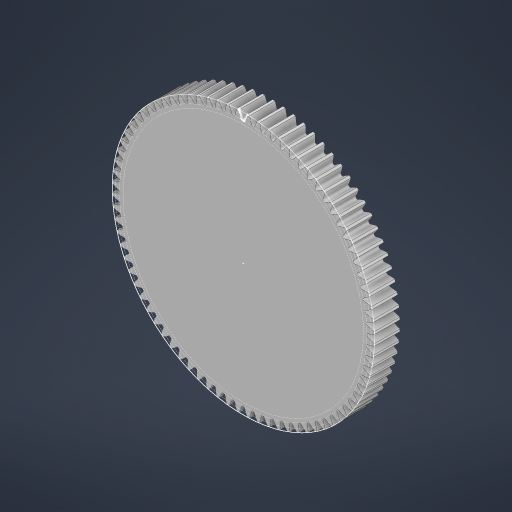
# Autodesk Inventor part: horizontal_axis_hal_gearr
Saved by Autodesk Inventor 2023.2 (Build 272271000, 271)
## iProperties
Created: 2023-07-30
Part Number: horizontal_axis_hal_gearr
Material: Generic
Document SubType Name: Modeling
Designer: Bober
Density: 1 g/cm^3
Appearance: Default
Author: Bober
Autodesk Inventor part; units mm, degrees
ref_plane "YZ Plane" through (0, 0, 0) normal (1, 0, 0) x (0, 1, 0)
ref_plane "XZ Plane" through (0, 0, 0) normal (0, 1, 0) x (-1, 0, 0)
ref_plane "XY Plane" through (0, 0, 0) normal (0, 0, 1) x (1, 0, 0)
sketch "Sketch1" plane through (0, 0, 0) normal (0, 0, 1) x (1, 0, 0)
  spline S0 degree 3 poles (-1.2376, 40.9813) (-1.1892, 40.8773) (-1.0925, 40.6692) (-0.9561, 40.3531) (-0.8267, 40.0342) (-0.7055, 39.712) (-0.5926, 39.3868) (-0.516, 39.1404) (-0.4674, 38.9752) (-0.4334, 38.8959) (-0.3865, 38.8233) (-0.3362, 38.7714) (-0.2894, 38.7381) (-0.2524, 38.7161) (-0.2127, 38.6991) (-0.1714, 38.6872) (-0.1291, 38.6784) (-0.0717, 38.676) (0, 38.6775) (0.0717, 38.676) (0.1291, 38.6784) (0.1714, 38.6872) (0.2127, 38.6991) (0.2524, 38.7161) (0.2894, 38.7381) (0.3362, 38.7714) (0.3865, 38.8233) (0.4334, 38.8959) (0.4674, 38.9752) (0.516, 39.1404) (0.5926, 39.3868) (0.7055, 39.712) (0.8267, 40.0342) (0.9561, 40.3531) (1.0925, 40.6692) (1.1892, 40.8773) (1.2376, 40.9813) knots 0 0 0 0 0.034418 0.068836 0.103253 0.137671 0.172089 0.206506 0.215109 0.223706 0.232301 0.240894 0.245196 0.249497 0.253799 0.2581 0.262401 0.266702 0.275307 0.283912 0.288213 0.292514 0.296815 0.301117 0.305418 0.30972 0.318313 0.326908 0.335505 0.344108 0.378525 0.412943 0.447361 0.481778 0.516196 0.550614 0.550614 0.550614 0.550614
  circle A0 centre (0, 0) radius 38.6769 construction
  circle A1 centre (0, 0) radius 37.5877 construction
  circle A2 centre (0, 0) radius 40 construction
  circle A3 centre (0, 0) radius 41
  point P0 (-1.0939, 40.6686)
  point P1 (-0.9573, 40.3527)
  point P2 (-0.8281, 40.0337)
  point P3 (-0.7069, 39.7115)
  point P4 (-0.5944, 39.3863)
  point P5 (-0.4918, 39.0577)
  point P6 (-0.4658, 38.9757)
  point P7 (-0.4313, 38.897)
  point P8 (-0.3843, 38.825)
  point P9 (-0.324, 38.7638)
  point P10 (-0.2891, 38.7386)
  point P11 (-0.252, 38.7169)
  point P12 (-0.2125, 38.6999)
  point P13 (-0.1712, 38.6877)
  point P14 (-0.129, 38.6796)
  point P15 (-0.086, 38.6769)
  point P16 (0, 38.6769)
  point P17 (0.086, 38.6769)
  point P18 (0.129, 38.6796)
  point P19 (0.1712, 38.6877)
  point P20 (0.2125, 38.6999)
  point P21 (0.252, 38.7169)
  point P22 (0.2891, 38.7386)
  point P23 (0.324, 38.7638)
  point P24 (0.3843, 38.825)
  point P25 (0.4313, 38.897)
  point P26 (0.4658, 38.9757)
  point P27 (0.4918, 39.0577)
  point P28 (0.5944, 39.3863)
  point P29 (0.7069, 39.7115)
  point P30 (0.8281, 40.0337)
  point P31 (0.9573, 40.3527)
  point P32 (1.0939, 40.6686)
  constraints: 4 centre point, 2 point on circle, 75 other
extrude "Extrusion1" add sketch "Sketch1" against normal blind 8
extrude "Extrusion2" cut sketch "Sketch1" against normal through all contours A3 S0 picked at (0.0203, 39.8707)
pattern_circular "Circular Pattern1" count 80 over 360 about axis through (0, 0, 0) along (0, 0, -1) of "Extrusion2"
equation "\"d0\" = FaceWidth"
equation "\"Module\" = 1"
equation "\"PressureAngle\" = 20deg"
equation "\"UnitProfileClearance\" = 0.25"
equation "\"UnitRoundRadius\" = 0.35"
equation "\"HeadDiameter\" = 82"
equation "\"RootDiameter\" = 77.35381"
equation "\"BaseDiameter\" = 75.17541"
equation "\"FaceWidth\" = 8"
equation "\"HelixAngle\" = 0"
equation "\"UnitCorrection\" = 0"
equation "\"UnitAddendumModification\" = 0"
equation "\"CircularPitch\" = 3.141593"
equation "\"UnitBacklashShift\" = -0.073095"
equation "\"TotalToolShift\" = -0.0731"
equation "\"IsInternal\" = 0"
body "Solid1"
